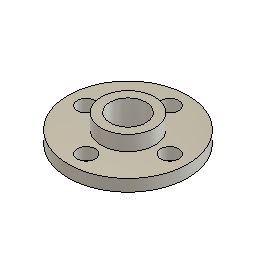
OmniWheel (Autodesk Fusion 360 archive; units mm, degrees)
design "25t servo horn"
Autodesk Fusion 360 part; units mm, degrees
sketch "Sketch1" plane through (0, 0, 0) normal (0, 1, 0) x (1, 0, 0)
  circle A0 centre (0, 0) radius 10
  circle A1 centre (0, 0) radius 4.5
  circle A2 centre (0, 0) radius 7 construction
  circle A3 centre (0, 0) radius 3
  line L0 (0, 0) -> (-10, 0) construction
  circle A4 centre (-7, 0) radius 1.5
  circle A5 centre (0, -7) radius 1.5
  circle A6 centre (7, 0) radius 1.5
  circle A7 centre (0, 7) radius 1.5
  dimension "d1" = 20
  dimension "d2" = 9
  dimension "d3" = 14
  dimension "d4" = 6
  dimension "d5" = 3
  dimension "d7" = 360
  constraint coincident A0.centre A1.centre
  constraint concentric A0 A1
  constraint concentric A1 A3
  constraint coincident A0 L0.end
  constraint horizontal L0
  constraint coincident L0 A4.centre
  constraint coincident A2 A4.centre
  measures "d1" diameter of A0
  measures "d2" diameter of A1
  measures "d3" diameter of A2
  measures "d4" diameter of A3
  measures "d5" diameter of A4
extrude "Extrude1" add sketch "Sketch1" along normal blind 2 contours A0
extrude "Extrude2" add sketch "Sketch1" along normal blind 4.5 contours A1

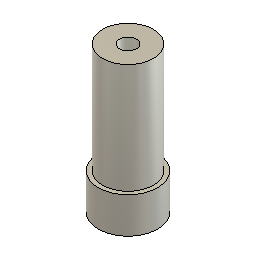
design "Coupler Omni"
Autodesk Fusion 360 part; units mm, degrees
sketch "Sketch1" plane through (0, 0, 0) normal (0, 1, 0) x (1, 0, 0)
  circle A0 centre (0, 0) radius 7
  circle A1 centre (0, 0) radius 2
  circle A2 centre (0, 0) radius 6
  dimension "d1" = 14
  dimension "d2" = 4
  dimension "d3" = 12
  constraint coincident A0.centre A1.centre
  constraint concentric A0 A1
  constraint concentric A0 A2
  measures "d1" diameter of A0
  measures "d2" diameter of A1
  measures "d3" diameter of A2
extrude "Extrude1" add sketch "Sketch1" along normal blind 8.5 contours A0 | A1 | A2
extrude "Extrude2" add sketch "Sketch1" along normal blind 23 contours A2
extrude "Extrude3" cut sketch "Sketch1" along normal blind 23 contours A1
extrude "Extrude4" add 1 faces at (4.6369, 23, 0.3974) along direction (0, 1, 0) blind 10.5
extrude "Extrude5" add 1 faces at (4.6369, 33.5, 0.3974) along direction (0, 1, 0) blind 1

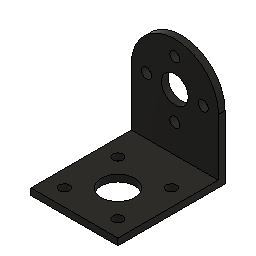
design "25mm Motor Mount"
Autodesk Fusion 360 part; units mm, degrees
sketch "Sketch1" plane through (0, 0, 0) normal (0, 0, 1) x (1, 0, 0)
  line L0 (0, 0) -> (26, 0)
  line L1 (26, 0) -> (26, 19)
  line L2 (0, 19) -> (0, 0)
  line L3 (0, 2) -> (26, 2)
  line L4 (13, 32) -> (13, 19) construction
  circle A0 centre (13, 19) radius 13
  circle A1 centre (13, 19) radius 4
  line L5 (13, 19) -> (26, 19) construction
  line L6 (13, 19) -> (0, 19) construction
  circle A2 centre (21.5, 19) radius 1.5
  circle A3 centre (4.5, 19) radius 1.5
  line L7 (13, 32) -> (0, 32) construction
  circle A4 centre (13, 10.5) radius 1.5
  circle A5 centre (13, 27.5) radius 1.5
  dimension "d1" = 26
  dimension "d3" = 2
  dimension "d4" = 13
  dimension "d5" = 26
  dimension "d6" = 8
  dimension "d7" = 3
  dimension "d8" = 8.5
  dimension "d9" = 3
  dimension "d10" = 8.5
  dimension "d11" = 32
  dimension "d28" = 90
  constraint horizontal L0
  constraint vertical L1
  constraint vertical L2
  constraint coincident L0.start L2.end
  constraint coincident L2 L3.start
  constraint coincident L1 L3.end
  constraint perpendicular L1 L3
  constraint coincident L4.end A0.centre
  constraint concentric A0 A1
  constraint coincident A0 L1.end
  constraint perpendicular L1 L5
  constraint perpendicular L4 L6
  constraint coincident L5 A2.centre
  constraint coincident L6 A3.centre
  constraint tangent A0 L7
  constraint perpendicular L4 L7
  measures "d1" distance of L0.start L0.end
  measures "d3" distance of L0 L3
  measures "d4" distance of L4.start L4.end
  measures "d5" diameter of A0
  measures "d6" diameter of A1
  measures "d7" diameter of A2
  measures "d8" distance of L4.end A2.centre
  measures "d9" diameter of A3
  measures "d10" distance of L4.end A3.centre
  measures "d11" distance of L0 L7
extrude "Extrude1" add sketch "Sketch1" along normal blind 2 contours L1 L2 L3 A0 | A0
extrude "Extrude2" add sketch "Sketch1" along normal blind 32 contours L0 L1 L2 L3
sketch "Sketch2" plane through (0, 2, 0) normal (0, 1, 0) x (-1, 0, 0)
  line L0 (-26, 2) -> (0, 2)
  line L1 (0, 2) -> (0, 32)
  line L2 (0, 32) -> (-26, 32)
  line L3 (-26, 32) -> (-26, 2)
  line L4 (-26, 19) -> (0, 19) construction
  circle A0 centre (-13, 19) radius 5
  line L5 (-26, 6) -> (0, 32) construction
  line L6 (0, 6) -> (-26, 32) construction
  line L7 (-21, 11) -> (-5, 11) construction
  line L8 (-26, 6) -> (0, 6) construction
  line L9 (-21, 11) -> (-21, 27) construction
  line L10 (-21, 27) -> (-5, 27) construction
  line L11 (-5, 11) -> (-5, 27) construction
  circle A1 centre (-5, 11) radius 1.5
  circle A2 centre (-21, 11) radius 1.5
  circle A3 centre (-21, 27) radius 1.5
  circle A4 centre (-5, 27) radius 1.5
  dimension "d16" = 10
  dimension "d17" = 16
  dimension "d18" = 26
  dimension "d19" = 13
  dimension "d20" = 26
  dimension "d21" = 3
  dimension "d22" = 3
  dimension "d23" = 3
  dimension "d24" = 3
  constraint midpoint L4 A0.centre
  constraint coincident L1.end L2.start
  constraint coincident L2.end L3.start
  constraint coincident L5 L7.start
  constraint coincident L6 L7.end
  constraint perpendicular L3 L7
  constraint coincident L1 L6.start
  constraint coincident L3 L5.start
  constraint coincident L3 L4.start
  constraint coincident L1 L4.end
  constraint coincident L6 L9.end
  constraint perpendicular L7 L9
  constraint coincident L5 L10.end
  constraint perpendicular L9 L10
  constraint coincident L7.end L11.start
  constraint coincident L7.start L9.start
  constraint coincident L9.end L10.start
  constraint coincident L10.end L11.end
  measures "d16" diameter of A0
  measures "d17" distance of L7.start L7.end
  measures "d18" distance of L1.end L6.start
  measures "d19" distance of L2 L4
  measures "d20" distance of L5.start L2.end
  measures "d21" diameter of A1
  measures "d22" diameter of A2
  measures "d23" diameter of A3
  measures "d24" diameter of A4
extrude "Extrude3" cut sketch "Sketch2" against normal blind 2 contours A0 | A1 | A2 | A3 | A4
